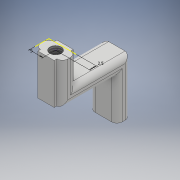
# Autodesk Inventor part: Lever
Saved by Autodesk Inventor 2017 (Build 210142000, 142)
## iProperties
Created: 2019-11-14
Part Number: Lever
Material: Generic
Document SubType Name: Modeling
Designer: kenli
Density: 1 g/cm^3
Appearance: Default
Author: kenli
Autodesk Inventor part; units mm, degrees
ref_plane "YZ Plane" through (0, 0, 0) normal (1, 0, 0) x (0, 1, 0)
ref_plane "XZ Plane" through (0, 0, 0) normal (0, 1, 0) x (-1, 0, 0)
ref_plane "XY Plane" through (0, 0, 0) normal (0, 0, 1) x (1, 0, 0)
sketch "Sketch1" plane through (0, 0, 0) normal (1, 0, 0) x (0, 1, 0)
  line L0 (0, 0) -> (0, -10)
  line L1 (0, -10) -> (20, -10)
  line L2 (20, -10) -> (20, -30)
  line L3 (20, -30) -> (15, -30)
  line L4 (15, -30) -> (15, -15)
  line L5 (15, -15) -> (-5, -15)
  line L6 (-5, -15) -> (-5, 0)
  line L7 (-5, 0) -> (0, 0)
  dimension "d0" = 10
  dimension "d1" = 20
  dimension "d2" = 20
  dimension "d3" = 5
  dimension "d4" = 15
  dimension "d5" = 20
  dimension "d6" = 15
  constraints: 16 end point, 5 perpendicular, 1 horizontal, 1 vertical
  measures "d0" distance of L0.start L0.end
  measures "d1" distance of L0.end L1.end
  measures "d2" distance of L1.end L2.end
  measures "d3" distance of L2.end L3.end
  measures "d4" distance of L3.end L4.end
  measures "d5" distance of L4.end L5.end
  measures "d6" distance of L5.end L6.end
extrude "Extrusion1" add sketch "Sketch1" along normal blind 10
sketch "Sketch2" plane through (0, -5, 0) normal (0, 0, 1) x (1, 0, 0)
  line L0 (0, 0) -> (0, 5) projected
  line L1 (0, 5) -> (10, 5) projected
  point P0 (5, 2.5)
  dimension "d9" = 5
  dimension "d10" = 2.5
  measures "d9" distance from line of point (5, 2.5) L0
  measures "d10" distance from line of point (5, 2.5) L1
sketch "Sketch3" plane through (0, -5, 0) normal (0, 0, 1) x (1, 0, 0)
  circle A0 centre (5, 2.5) radius 2.0828
  line L0 (10, 5) -> (10, 0) projected
  line L1 (0, 5) -> (10, 5) projected
  dimension "d11" = 4.1656
  dimension "d12" = 5
  dimension "d13" = 2.5
  constraints: 1 centre point
  measures "d11" diameter of A0
  measures "d12" distance from line of L0 A0.centre
  measures "d13" distance from line of A0.centre L1
extrude "Extrusion2" cut sketch "Sketch3" against normal blind 10
thread "Thread1" size "8-32 UNC" class "2B" standard "ANSI Unified Screw Threads" full length
fillet "Fillet1" radius 2 12 edges at (10, 20, -20) (0, 20, -20) (10, 0, -5) (0, 0, -5) (10, 15, -22.5) (10, -5, -7.5) (0, -5, -7.5) (0, 10, -10) (0, 5, -15) (10, 10, -10) (0, 15, -22.5) (10, 5, -15)
sketch "Sketch4" plane through (2, -5, -15) normal (0, -1, 0) x (1, 0, 0)
  line L0 (0, 15) -> (0, 5) projected
  line L1 (6, -15) -> (6, 5) projected
  line L2 (0, 15) -> (6, 15)
  line L3 (6, 15) -> (6, 0.0408)
  line L4 (6, 0.0408) -> (0, 0.0408)
  line L5 (0, 0.0408) -> (0, 15)
  point P0 (-2, 15)
  constraints: 8 end point, 2 parallel, 1 horizontal, 1 perpendicular, 1 point on line
extrude "Extrusion3" add sketch "Sketch4" along normal blind 1
sketch "Sketch5" plane through (2, 0, 0) normal (0, 1, 0) x (1, 0, 0)
  line L0 (6, 10) -> (6, 0) projected
  line L1 (0, 10) -> (6, 10) projected
  line L2 (6, 0) -> (0, 0)
  line L3 (0, 0) -> (0, 10)
  line L4 (0, 10) -> (6, 10)
  line L5 (6, 10) -> (6, 0)
  point P0 (-2, 0)
  constraints: 8 end point, 2 parallel, 1 horizontal, 1 perpendicular
extrude "Extrusion4" add sketch "Sketch5" along normal blind 1
body "Solid1"
